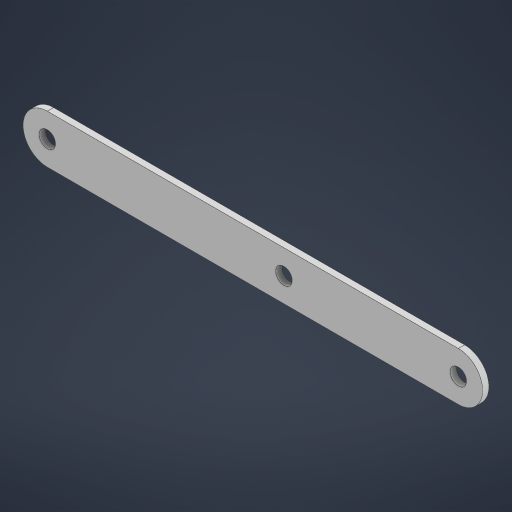
# Autodesk Inventor part: ArmConnector2Mini
Saved by Autodesk Inventor 2024.2 (Build 282272000, 272)
## iProperties
Created: 2024-01-19
Part Number: ArmConnector2Mini
Material: Generic
Document SubType Name: Modeling
Designer: ctam0
Density: 1 g/cm^3
Appearance: Default
Author: ctam0
Autodesk Inventor part; units mm, degrees
ref_plane "YZ Plane" through (0, 0, 0) normal (1, 0, 0) x (0, 1, 0)
ref_plane "XZ Plane" through (0, 0, 0) normal (0, 1, 0) x (-1, 0, 0)
ref_plane "XY Plane" through (0, 0, 0) normal (0, 0, 1) x (1, 0, 0)
sketch "Sketch1" plane through (0, 0, 0) normal (0, 0, 1) x (1, 0, 0)
  line L0 (-33.1724, -3.9116) -> (33.1724, -3.9116)
  line L1 (33.1724, 3.9116) -> (-33.1724, 3.9116)
  line L2 (-33.1724, -3.9116) -> (33.1724, 3.9116) construction
  line L3 (33.1724, -3.9116) -> (-33.1724, 3.9116) construction
  arc A0 (-33.1724, 3.9116) -> (-33.134, -3.9114) centre (-33.1724, 0) ccw
  arc A1 (33.1724, -3.9116) -> (33.1724, 3.9116) centre (33.1724, 0) ccw
  circle A2 centre (-33.1724, 0) radius 1.3208
  circle A3 centre (5.0292, 0) radius 1.3208
  circle A4 centre (33.1724, 0) radius 1.3208
  point P0 (0, 0)
  dimension "d2" = 2.6416
  dimension "d3" = 2.6416
  dimension "d4" = 2.6416
  dimension "d5" = 35.56
  constraints: 8 end point, 5 centre point, 4 point on circle, 2 coincident, 2 midpoint, 1 horizontal, 1 parallel
  measures "d2" diameter of A2
  measures "d3" diameter of A3
  measures "d4" diameter of A4
extrude "Extrusion1" add sketch "Sketch1" along normal blind 1.016
body "Solid1"
